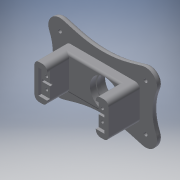
# Autodesk Inventor part: уменьшанная версия блока подшипников
Saved by Autodesk Inventor 2019.1 (Build 231200000, 200)
## iProperties
Created: 2018-09-01
Part Number: уменьшанная версия блока подшипников
Material: Типовые
Document SubType Name: Modeling
Designer: Олег
Density: 1 g/cm^3
Appearance: По умолчанию
Author: Олег
Autodesk Inventor part; units mm, degrees
ref_plane "YZ Plane" through (0, 0, 0) normal (1, 0, 0) x (0, 1, 0)
ref_plane "XZ Plane" through (0, 0, 0) normal (0, 1, 0) x (-1, 0, 0)
ref_plane "XY Plane" through (0, 0, 0) normal (0, 0, 1) x (1, 0, 0)
sketch "Эскиз1" plane through (0, 0, 0) normal (0, 0, 1) x (1, 0, 0)
  line L0 (32, -15) -> (-32, -15)
  line L1 (-32, -15) -> (-32, 15)
  line L2 (-32, 15) -> (32, 15)
  line L3 (32, 15) -> (32, -15)
  line L4 (32, -15) -> (-32, 15) construction
  line L5 (-32, -15) -> (32, 15) construction
  line L6 (24, -5) -> (-24, -5) construction
  line L7 (-24, -5) -> (-24, 5) construction
  line L8 (-24, 5) -> (24, 5) construction
  line L9 (24, 5) -> (24, -5) construction
  line L10 (24, -5) -> (-24, 5) construction
  line L11 (-24, -5) -> (24, 5) construction
  circle A0 centre (10, 0) radius 13.075
  point P0 (0, 0)
  point P1 (0, 0)
  dimension "d0" = 64
  dimension "d1" = 30
  dimension "d2" = 48
  dimension "d3" = 10
  dimension "d4" = 26.15
  dimension "d5" = 14
  constraints: 24 end point, 5 midpoint, 4 parallel, 2 horizontal, 2 perpendicular, 1 centre point, 1 horizontal alignment
  measures "d0" distance of L1.end L2.end
  measures "d1" distance of L0.end L1.end
  measures "d2" distance of L7.end L8.end
  measures "d3" distance of L6.end L7.end
  measures "d4" diameter of A0
  measures "d5" distance from line of L9 A0.centre
extrude "Выдавливание1" add sketch "Эскиз1" along normal blind 13
ref_plane "РабПлоскость1" through (0, 0, 5) normal (0, 0, -1) x (-1, 0, 0)
sketch "Эскиз2" plane through (0, 0, 5) normal (0, 0, -1) x (-1, 0, 0)
  circle A0 centre (-10, 0) radius 13.075 projected
  circle A1 centre (-10, 0) radius 12.075
  point P0 (0, 0)
  dimension "d9" = 1
  constraints: 1 centre point
  measures "d9" radial gap between concentric circles of A0 A1
extrude "Выдавливание2" add sketch "Эскиз2" against normal blind 3
sketch "Эскиз3" plane through (0, 0, 13) normal (0, 0, 1) x (1, 0, 0)
  line L0 (32, 15) -> (-32, 15) projected
  line L1 (-32, -15) -> (32, -15) projected
  line L2 (-32, 15) -> (-21, 15)
  line L3 (-21, 15) -> (-21, -15)
  line L4 (-21, -15) -> (-32, -15)
  line L5 (-32, -15) -> (-32, 15)
  line L6 (32, -15) -> (32, 15) projected
  line L7 (32, 15) -> (21, 15)
  line L8 (21, 15) -> (21, -15)
  line L9 (21, -15) -> (32, -15)
  line L10 (32, -15) -> (32, 15)
  point P0 (0, 0)
  dimension "d12" = 42
  dimension "d13" = 21
  constraints: 16 end point, 4 parallel, 2 horizontal, 2 perpendicular, 2 point on line
  measures "d12" distance between parallel lines of L3 L8
  measures "d13" distance from line of point (0, 0) L8
extrude "Выдавливание3" add sketch "Эскиз3" along normal blind 19 contours L6 L1 L8 L0 | L3 L1 L5 L0
sketch "Эскиз4" plane through (0, 0, 32) normal (0, 0, 1) x (1, 0, 0)
  line L0 (-20, 10.5) -> (-28, 10.5)
  line L1 (-28, 10.5) -> (-28, -10.5)
  line L2 (-28, -10.5) -> (-20, -10.5)
  line L3 (-20, -10.5) -> (-20, 10.5)
  line L4 (-20, 10.5) -> (-28, -10.5) construction
  line L5 (-28, 10.5) -> (-20, -10.5) construction
  line L6 (28, -10.5) -> (20, -10.5)
  line L7 (20, -10.5) -> (20, 10.5)
  line L8 (20, 10.5) -> (28, 10.5)
  line L9 (28, 10.5) -> (28, -10.5)
  line L10 (28, -10.5) -> (20, 10.5) construction
  line L11 (20, -10.5) -> (28, 10.5) construction
  point P0 (0, 0)
  point P1 (-24, 0)
  point P2 (-24, 0)
  point P3 (24, 0)
  point P4 (24, 0)
  dimension "d16" = 8
  dimension "d17" = 21
  dimension "d18" = 20
  dimension "d19" = 8
  dimension "d20" = 21
  dimension "d21" = 20
  constraints: 24 end point, 6 midpoint, 4 parallel, 2 horizontal, 2 horizontal alignment, 2 perpendicular
  measures "d16" distance of L2.end L1.end
  measures "d17" distance of L1.end L0.end
  measures "d18" distance from line of point (0, 0) L3
  measures "d19" distance of L7.end L8.end
  measures "d20" distance of L6.end L7.end
  measures "d21" distance from line of point (0, 0) L7
extrude "Выдавливание4" cut sketch "Эскиз4" against normal blind 2.6
sketch "Эскиз5" plane through (0, 0, 0) normal (0, 0, -1) x (-1, 0, 0)
  line L0 (-32, 15) -> (-32, -15) projected
  line L1 (-32, -15) -> (32, -15) projected
  line L2 (32, 15) -> (-32, 15) projected
  line L3 (32, -15) -> (32, 15) projected
  line L4 (-37, 20) -> (37, 20)
  line L5 (37, 20) -> (37, -20)
  line L6 (37, -20) -> (-37, -20)
  line L7 (-37, -20) -> (-37, 20)
  line L8 (-37, 20) -> (37, -20) construction
  line L9 (37, 20) -> (-37, -20) construction
  point P0 (0, 0)
  dimension "d24" = 74
  dimension "d25" = 40
  constraints: 12 end point, 2 midpoint, 2 parallel, 1 horizontal, 1 perpendicular
  measures "d24" distance of L5.end L6.end
  measures "d25" distance of L4.end L5.end
extrude "Выдавливание5" add sketch "Эскиз5" against normal blind 5
sketch "Эскиз6" plane through (0, 0, 0) normal (0, 0, -1) x (-1, 0, 0)
  line L0 (-37, 20) -> (37, 20) projected
  circle A0 centre (37, 20) radius 10
  line L1 (37, -20) -> (-37, -20) projected
  circle A1 centre (37, -20) radius 10
  circle A2 centre (-37, -20) radius 10
  line L2 (0, -20) -> (-34.2973, -29.6278)
  line L3 (0, -20) -> (34.2973, -29.6278)
  line L4 (0, 20) -> (34.2973, 29.6278)
  line L5 (-37, -20) -> (-37, 20) projected
  circle A3 centre (-37, 20) radius 10
  line L6 (0, 20) -> (-34.2973, 29.6278)
  line L7 (-37, 0) -> (-45.6603, -15)
  line L8 (-37, 0) -> (-45.6603, 15)
  line L9 (37, 20) -> (37, -20) projected
  line L10 (37, 0) -> (45.6603, -15)
  line L11 (37, 0) -> (45.6603, 15)
  point P0 (0, 0)
  dimension "d28" = 20
  dimension "d29" = 20
  dimension "d30" = 20
  dimension "d32" = 20
  constraints: 16 end point, 8 point on circle, 8 tangent, 4 centre point, 4 midpoint, 2 coincident
  measures "d28" diameter of A0
  measures "d29" diameter of A1
  measures "d30" diameter of A2
  measures "d32" diameter of A3
extrude "Выдавливание6" add sketch "Эскиз6" against normal blind 5 contours L5 A3 L0 | A3 L6 L0 | L5 L8 A3 | L4 A0 L0 | L5 A2 L7 | A0 L9 L0 | L5 L1 A2 | A0 L11 L9 | L1 L2 A2 | L10 A1 L9 | L1 A1 L3 | A1 L1 L9 picked at (-43.0839, 17.3904) picked at (41.5807, 24.7826) picked at (-43.0839, -17.3904) picked at (40.3666, -25.7029)
sketch "Эскиз7" plane through (0, 0, 0) normal (0, 0, -1) x (-1, 0, 0)
  arc A0 (34.2973, -29.6278) -> (45.6603, -15) centre (37, -20) ccw projected
  arc A1 (45.6603, 15) -> (34.2973, 29.6278) centre (37, 20) ccw projected
  arc A2 (-34.2973, 29.6278) -> (-45.6603, 15) centre (-37, 20) ccw projected
  arc A3 (-45.6603, -15) -> (-34.2973, -29.6278) centre (-37, -20) ccw projected
  circle A4 centre (-37, -20) radius 1.6
  circle A5 centre (-37, 20) radius 1.6
  circle A6 centre (37, 20) radius 1.6
  circle A7 centre (37, -20) radius 1.6
  point P0 (0, 0)
  dimension "d35" = 3.2
  dimension "d36" = 3.2
  dimension "d37" = 3.2
  dimension "d38" = 3.2
  constraints: 4 centre point, 4 coincident
  measures "d35" diameter of A4
  measures "d36" diameter of A5
  measures "d37" diameter of A6
  measures "d38" diameter of A7
extrude "Выдавливание7" cut sketch "Эскиз7" against normal blind 5
chamfer "Фаска1" distance 2 angle 45 4 edges at (38.6, -20, 0) (38.6, 20, 0) (-35.4, 20, 0) (-35.4, -20, 0)
fillet "Сопряжение1" radius 85 2 edges at (0, -20, 2.5) (0, 20, 2.5)
fillet "Сопряжение2" radius 42 2 edges at (37, 0, 2.5) (-37, 0, 2.5)
sketch "Эскиз8" plane through (0, 0, 29.4) normal (0, 0, 1) x (1, 0, 0)
  line L0 (-24, 5) -> (24, 5) construction
  line L1 (24, 5) -> (24, -5) construction
  line L2 (24, -5) -> (-24, -5) construction
  line L3 (-24, -5) -> (-24, 5) construction
  line L4 (-24, 5) -> (24, -5) construction
  line L5 (24, 5) -> (-24, -5) construction
  circle A0 centre (24, -5) radius 1.25
  circle A1 centre (24, 5) radius 1.25
  circle A2 centre (-24, -5) radius 1.25
  circle A3 centre (-24, 5) radius 1.25
  line L6 (20, 1) -> (28, 1)
  line L7 (28, 1) -> (28, -1)
  line L8 (28, -1) -> (20, -1)
  line L9 (20, -1) -> (20, 1)
  line L10 (20, 1) -> (28, -1) construction
  line L11 (28, 1) -> (20, -1) construction
  line L12 (-28, 1) -> (-20, 1)
  line L13 (-20, 1) -> (-20, -1)
  line L14 (-20, -1) -> (-28, -1)
  line L15 (-28, -1) -> (-28, 1)
  line L16 (-28, 1) -> (-20, -1) construction
  line L17 (-20, 1) -> (-28, -1) construction
  point P0 (0, 0)
  point P1 (24, 0)
  point P2 (-24, 0)
  dimension "d46" = 48
  dimension "d47" = 10
  dimension "d48" = 2.5
  dimension "d49" = 2.5
  dimension "d50" = 2.5
  dimension "d51" = 2.5
  dimension "d52" = 8
  dimension "d53" = 2
  dimension "d54" = 8
  dimension "d55" = 2
  constraints: 36 end point, 8 midpoint, 6 parallel, 4 centre point, 4 coincident, 3 horizontal, 3 perpendicular
  measures "d46" distance of L1.end L2.end
  measures "d47" distance of L0.end L1.end
  measures "d48" diameter of A0
  measures "d49" diameter of A1
  measures "d50" diameter of A2
  measures "d51" diameter of A3
  measures "d52" distance of L7.end L8.end
  measures "d53" distance of L6.end L7.end
  measures "d54" distance of L13.end L14.end
  measures "d55" distance of L12.end L13.end
extrude "Выдавливание8" cut sketch "Эскиз8" against normal blind 2
sketch "Эскиз9" plane through (24, 5, 27.4) normal (0, 0, 1) x (1, 0, 0)
  circle A0 centre (0, 0) radius 1.25 projected
  circle A1 centre (0, -10) radius 1.25 projected
  circle A2 centre (-48, -10) radius 1.25 projected
  circle A3 centre (-48, 0) radius 1.25 projected
  point P0 (-24, -5)
extrude "Выдавливание9" cut sketch "Эскиз9" against normal blind 10
sketch "Эскиз10" plane through (10, 0, 8) normal (0, 0, 1) x (1, 0, 0)
  circle A0 centre (0, 0) radius 12.075 projected
  circle A1 centre (0, 0) radius 13.075 projected
  point P0 (-10, 0)
extrude "Выдавливание10" cut sketch "Эскиз10" along normal blind 14 contours A0 | A1
fillet "Сопряжение3" radius 3 2 edges at (22.5455, 3.6831, 22) (22.5455, -3.6831, 22)
fillet "Сопряжение4" radius 3 12 edges at (-28.6351, 28.0384, 0) (-44.4861, 26.6302, 0) (-43, 0, 0) (-44.4861, -26.6302, 0) (-28.6351, -28.0384, 0) (0, -23.2856, 0) (28.6351, -28.0384, 0) (44.4861, -26.6302, 0) (43, 0, 0) (44.4861, 26.6302, 0) (28.6351, 28.0384, 0) (0, 23.2856, 0)
fillet "Сопряжение5" radius 4 4 edges at (32, 15, 18.5) (32, -15, 18.5) (-32, -15, 18.5) (-32, 15, 18.5)
fillet "Сопряжение6" radius 4 4 edges at (21, 15, 22.5) (21, -15, 22.5) (-21, -15, 22.5) (-21, 15, 22.5)
fillet "Сопряжение7" radius 2 6 edges at (-23, 15, 13) (0, 15, 13) (23, 15, 13) (23, -15, 13) (0, -15, 13) (-23, -15, 13)
sketch "Эскиз11" plane through (0, 0, 32) normal (0, 0, 1) x (1, 0, 0)
  line L0 (-28, 1) -> (-28, 10.5) projected
  line L1 (-28, 10.5) -> (-28.5, 10.5)
  line L2 (-28.5, 10.5) -> (-28.5, -10.5)
  line L3 (-28.5, -10.5) -> (-28, -10.5)
  line L4 (-28, -10.5) -> (-28, 10.5)
  line L5 (28, 10.5) -> (28.5, 10.5)
  line L6 (28.5, 10.5) -> (28.5, -10.5)
  line L7 (28.5, -10.5) -> (28, -10.5)
  line L8 (28, -10.5) -> (28, 10.5)
  point P0 (0, 0)
  dimension "d67" = 0.5
  dimension "d68" = 0.5
  dimension "d69" = 21
  dimension "d70" = 21
  constraints: 16 end point, 4 parallel, 2 horizontal, 2 perpendicular
  measures "d67" distance of L3.end L2.end
  measures "d68" distance of L6.end L7.end
  measures "d69" distance of L5.end L6.end
  measures "d70" distance of L1.end L2.end
extrude "Выдавливание11" cut sketch "Эскиз11" against normal up to surface (2.6 mm away)
equation "\"d28\" = d29"
equation "\"d30\" = d29"
equation "\"d32\" = d28"
equation "\"d49\" = d48"
equation "\"d50\" = d48"
equation "\"d51\" = d50"
